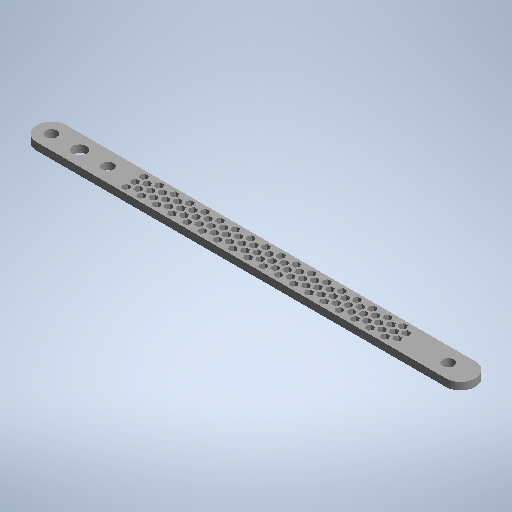
# Autodesk Inventor part: RT_ARM_PR_001
Saved by Autodesk Inventor 2025.4 (Build 294407000, 407)
## iProperties
Created: 2026-04-27
Part Number: RT_ARM_PR_001
Material: Générique
Document SubType Name: Modeling
Designer: louis
Density: 1 g/cm^3
Appearance: Par défaut
Author: louis
Autodesk Inventor part; units mm, degrees
ref_plane "YZ Plane" through (0, 0, 0) normal (1, 0, 0) x (0, 1, 0)
ref_plane "XZ Plane" through (0, 0, 0) normal (0, 1, 0) x (-1, 0, 0)
ref_plane "XY Plane" through (0, 0, 0) normal (0, 0, 1) x (1, 0, 0)
sketch "Sketch2" plane through (0, 0, 0) normal (0, 0, 1) x (1, 0, 0)
  line L0 (-89.25, 6) -> (89.25, 6)
  line L1 (89.25, 6) -> (89.25, -6)
  line L2 (89.25, -6) -> (-89.25, -6)
  line L3 (-89.25, -6) -> (-89.25, 6)
  line L4 (-89.25, 6) -> (89.25, -6) construction
  line L5 (89.25, 6) -> (-89.25, -6) construction
  line L6 (-83.25, 0) -> (-60.25, 0) construction
  line L7 (-83.25, -6) -> (-60.25, -6)
  line L8 (-60.25, 6) -> (-83.25, 6)
  arc A0 (-83.25, 6) -> (-83.25, -6) centre (-83.25, 0) ccw
  arc A1 (-60.25, -6) -> (-60.25, 6) centre (-60.25, 0) ccw
  line L9 (73.25, 0) -> (83.25, 0) construction
  line L10 (73.25, -6) -> (83.25, -6)
  line L11 (83.25, 6) -> (73.25, 6)
  arc A2 (73.25, 6) -> (73.25, -6) centre (73.25, 0) ccw
  arc A3 (83.25, -6) -> (83.25, 6) centre (83.25, 0) ccw
  line L12 (-47.75, 0) -> (-48.5, -1.299)
  line L13 (-48.5, -1.299) -> (-50, -1.299)
  line L14 (-50, -1.299) -> (-50.75, 0)
  line L15 (-50.75, 0) -> (-50, 1.299)
  line L16 (-50, 1.299) -> (-48.5, 1.299)
  line L17 (-48.5, 1.299) -> (-47.75, 0)
  line L18 (-47.75, 3.5981) -> (-48.5, 2.299)
  line L19 (-48.5, 2.299) -> (-50, 2.299)
  line L20 (-50, 2.299) -> (-50.75, 3.5981)
  line L21 (-50.75, 3.5981) -> (-50, 4.8971)
  line L22 (-50, 4.8971) -> (-48.5, 4.8971)
  line L23 (-48.5, 4.8971) -> (-47.75, 3.5981)
  line L24 (-50, 1.299) -> (-50, 2.299) construction
  line L25 (-45.384, 0.5) -> (-46.884, 0.5)
  line L26 (-46.884, 0.5) -> (-47.634, 1.799)
  line L27 (-47.634, 1.799) -> (-46.884, 3.0981)
  line L28 (-46.884, 3.0981) -> (-45.384, 3.0981)
  line L29 (-45.384, 3.0981) -> (-44.634, 1.799)
  line L30 (-44.634, 1.799) -> (-45.384, 0.5)
  line L31 (-48.5, -4.8971) -> (-50, -4.8971)
  line L32 (-50, -4.8971) -> (-50.75, -3.5981)
  line L33 (-50.75, -3.5981) -> (-50, -2.299)
  line L34 (-50, -2.299) -> (-48.5, -2.299)
  line L35 (-48.5, -2.299) -> (-47.75, -3.5981)
  line L36 (-47.75, -3.5981) -> (-48.5, -4.8971)
  line L37 (-44.634, -1.799) -> (-45.384, -3.0981)
  line L38 (-45.384, -3.0981) -> (-46.884, -3.0981)
  line L39 (-46.884, -3.0981) -> (-47.634, -1.799)
  line L40 (-47.634, -1.799) -> (-46.884, -0.5)
  line L41 (-46.884, -0.5) -> (-45.384, -0.5)
  line L42 (-45.384, -0.5) -> (-44.634, -1.799)
  line L43 (-50, -1.299) -> (-50, -2.299) construction
  line L44 (-44.634, 1.799) -> (-43.7679, 2.299) construction
  line L45 (-43.7679, 2.299) -> (-43.7679, 1.299) construction
  line L46 (-43.7679, 1.299) -> (-44.634, 1.799) construction
  line L47 (-43.7679, 1.299) -> (-44.5179, 0) construction
  line L48 (-44.5179, 0) -> (-45.384, 0.5) construction
  line L49 (-45.384, -0.5) -> (-44.5179, 0) construction
  line L50 (-50.75, 3.5981) -> (-50.75, 0) construction
  line L51 (-44.55, 3.5981) -> (-44.55, 0) construction
  line L52 (-44.55, 0) -> (-43.8, 1.299)
  line L53 (-44.55, 3.5981) -> (-43.8, 4.8971)
  line L54 (-43.8, 2.299) -> (-44.55, 3.5981)
  line L55 (-43.8, 1.299) -> (-43.8, 2.299) construction
  line L56 (-42.3, 2.299) -> (-43.8, 2.299)
  line L57 (-43.8, 4.8971) -> (-42.3, 4.8971)
  line L58 (-43.8, 1.299) -> (-42.3, 1.299)
  line L59 (-42.3, 1.299) -> (-41.55, 0)
  line L60 (-41.55, 3.5981) -> (-42.3, 2.299)
  line L61 (-40.684, 0.5) -> (-41.434, 1.799)
  line L62 (-41.434, 1.799) -> (-40.684, 3.0981)
  line L63 (-42.3, 4.8971) -> (-41.55, 3.5981)
  line L64 (-41.55, 0) -> (-42.3, -1.299)
  line L65 (-42.3, -1.299) -> (-43.8, -1.299)
  line L66 (-43.8, -1.299) -> (-44.55, 0)
  line L67 (-43.8, -1.299) -> (-43.8, -2.299) construction
  line L68 (-43.8, -2.299) -> (-42.3, -2.299)
  line L69 (-40.684, -3.0981) -> (-41.434, -1.799)
  line L70 (-44.55, -3.5981) -> (-43.8, -2.299)
  line L71 (-42.3, -2.299) -> (-41.55, -3.5981)
  line L72 (-43.8, -4.8971) -> (-44.55, -3.5981)
  line L73 (-42.3, -4.8971) -> (-43.8, -4.8971)
  line L74 (-41.55, -3.5981) -> (-42.3, -4.8971)
  line L75 (-41.434, -1.799) -> (-40.684, -0.5)
  line L76 (-38.3179, 0) -> (-39.184, 0.5) construction
  line L77 (-39.184, -0.5) -> (-38.3179, 0) construction
  line L78 (-39.184, 3.0981) -> (-38.434, 1.799)
  line L79 (-38.434, 1.799) -> (-39.184, 0.5)
  line L80 (-38.434, -1.799) -> (-39.184, -3.0981)
  line L81 (-39.184, -0.5) -> (-38.434, -1.799)
  line L82 (-39.184, -3.0981) -> (-40.684, -3.0981)
  line L83 (-40.684, -0.5) -> (-39.184, -0.5)
  line L84 (-39.184, 0.5) -> (-40.684, 0.5)
  line L85 (-40.684, 3.0981) -> (-39.184, 3.0981)
  line L86 (-38.35, 3.5981) -> (-38.35, 0) construction
  line L87 (-38.35, 0) -> (-37.6, 1.299)
  line L88 (-38.35, 3.5981) -> (-37.6, 4.8971)
  line L89 (-37.6, 2.299) -> (-38.35, 3.5981)
  line L90 (-37.6, 1.299) -> (-37.6, 2.299) construction
  line L91 (-36.1, 2.299) -> (-37.6, 2.299)
  line L92 (-37.6, 4.8971) -> (-36.1, 4.8971)
  line L93 (-37.6, 1.299) -> (-36.1, 1.299)
  line L94 (-36.1, 1.299) -> (-35.35, 0)
  line L95 (-35.35, 3.5981) -> (-36.1, 2.299)
  line L96 (-34.484, 0.5) -> (-35.234, 1.799)
  line L97 (-35.234, 1.799) -> (-34.484, 3.0981)
  line L98 (-36.1, 4.8971) -> (-35.35, 3.5981)
  line L99 (-35.35, 0) -> (-36.1, -1.299)
  line L100 (-36.1, -1.299) -> (-37.6, -1.299)
  line L101 (-37.6, -1.299) -> (-38.35, 0)
  line L102 (-37.6, -1.299) -> (-37.6, -2.299) construction
  line L103 (-37.6, -2.299) -> (-36.1, -2.299)
  line L104 (-34.484, -3.0981) -> (-35.234, -1.799)
  line L105 (-38.35, -3.5981) -> (-37.6, -2.299)
  line L106 (-36.1, -2.299) -> (-35.35, -3.5981)
  line L107 (-37.6, -4.8971) -> (-38.35, -3.5981)
  line L108 (-36.1, -4.8971) -> (-37.6, -4.8971)
  line L109 (-35.35, -3.5981) -> (-36.1, -4.8971)
  line L110 (-35.234, -1.799) -> (-34.484, -0.5)
  line L111 (-32.1179, 0) -> (-32.984, 0.5) construction
  line L112 (-32.984, -0.5) -> (-32.1179, 0) construction
  line L113 (-32.984, 3.0981) -> (-32.234, 1.799)
  line L114 (-32.234, 1.799) -> (-32.984, 0.5)
  line L115 (-32.234, -1.799) -> (-32.984, -3.0981)
  line L116 (-32.984, -0.5) -> (-32.234, -1.799)
  line L117 (-32.984, -3.0981) -> (-34.484, -3.0981)
  line L118 (-34.484, -0.5) -> (-32.984, -0.5)
  line L119 (-32.984, 0.5) -> (-34.484, 0.5)
  line L120 (-34.484, 3.0981) -> (-32.984, 3.0981)
  line L121 (-32.15, 3.5981) -> (-32.15, 0) construction
  line L122 (-32.15, 0) -> (-31.4, 1.299)
  line L123 (-32.15, 3.5981) -> (-31.4, 4.8971)
  line L124 (-31.4, 2.299) -> (-32.15, 3.5981)
  line L125 (-31.4, 1.299) -> (-31.4, 2.299) construction
  line L126 (-29.9, 2.299) -> (-31.4, 2.299)
  line L127 (-31.4, 4.8971) -> (-29.9, 4.8971)
  line L128 (-31.4, 1.299) -> (-29.9, 1.299)
  line L129 (-29.9, 1.299) -> (-29.15, 0)
  line L130 (-29.15, 3.5981) -> (-29.9, 2.299)
  line L131 (-28.284, 0.5) -> (-29.034, 1.799)
  line L132 (-29.034, 1.799) -> (-28.284, 3.0981)
  line L133 (-29.9, 4.8971) -> (-29.15, 3.5981)
  line L134 (-29.15, 0) -> (-29.9, -1.299)
  line L135 (-29.9, -1.299) -> (-31.4, -1.299)
  line L136 (-31.4, -1.299) -> (-32.15, 0)
  line L137 (-31.4, -1.299) -> (-31.4, -2.299) construction
  line L138 (-31.4, -2.299) -> (-29.9, -2.299)
  line L139 (-28.284, -3.0981) -> (-29.034, -1.799)
  line L140 (-32.15, -3.5981) -> (-31.4, -2.299)
  line L141 (-29.9, -2.299) -> (-29.15, -3.5981)
  line L142 (-31.4, -4.8971) -> (-32.15, -3.5981)
  line L143 (-29.9, -4.8971) -> (-31.4, -4.8971)
  line L144 (-29.15, -3.5981) -> (-29.9, -4.8971)
  line L145 (-29.034, -1.799) -> (-28.284, -0.5)
  line L146 (-25.9179, 0) -> (-26.784, 0.5) construction
  line L147 (-26.784, -0.5) -> (-25.9179, 0) construction
  line L148 (-26.784, 3.0981) -> (-26.034, 1.799)
  line L149 (-26.034, 1.799) -> (-26.784, 0.5)
  line L150 (-26.034, -1.799) -> (-26.784, -3.0981)
  line L151 (-26.784, -0.5) -> (-26.034, -1.799)
  line L152 (-26.784, -3.0981) -> (-28.284, -3.0981)
  line L153 (-28.284, -0.5) -> (-26.784, -0.5)
  line L154 (-26.784, 0.5) -> (-28.284, 0.5)
  line L155 (-28.284, 3.0981) -> (-26.784, 3.0981)
  line L156 (-25.95, 3.5981) -> (-25.95, 0) construction
  line L157 (-25.95, 0) -> (-25.2, 1.299)
  line L158 (-25.95, 3.5981) -> (-25.2, 4.8971)
  line L159 (-25.2, 2.299) -> (-25.95, 3.5981)
  line L160 (-25.2, 1.299) -> (-25.2, 2.299) construction
  line L161 (-23.7, 2.299) -> (-25.2, 2.299)
  line L162 (-25.2, 4.8971) -> (-23.7, 4.8971)
  line L163 (-25.2, 1.299) -> (-23.7, 1.299)
  line L164 (-23.7, 1.299) -> (-22.95, 0)
  line L165 (-22.95, 3.5981) -> (-23.7, 2.299)
  line L166 (-22.084, 0.5) -> (-22.834, 1.799)
  line L167 (-22.834, 1.799) -> (-22.084, 3.0981)
  line L168 (-23.7, 4.8971) -> (-22.95, 3.5981)
  line L169 (-22.95, 0) -> (-23.7, -1.299)
  line L170 (-23.7, -1.299) -> (-25.2, -1.299)
  line L171 (-25.2, -1.299) -> (-25.95, 0)
  line L172 (-25.2, -1.299) -> (-25.2, -2.299) construction
  line L173 (-25.2, -2.299) -> (-23.7, -2.299)
  line L174 (-22.084, -3.0981) -> (-22.834, -1.799)
  line L175 (-25.95, -3.5981) -> (-25.2, -2.299)
  line L176 (-23.7, -2.299) -> (-22.95, -3.5981)
  line L177 (-25.2, -4.8971) -> (-25.95, -3.5981)
  line L178 (-23.7, -4.8971) -> (-25.2, -4.8971)
  line L179 (-22.95, -3.5981) -> (-23.7, -4.8971)
  line L180 (-22.834, -1.799) -> (-22.084, -0.5)
  line L181 (-19.7179, 0) -> (-20.584, 0.5) construction
  line L182 (-20.584, -0.5) -> (-19.7179, 0) construction
  line L183 (-20.584, 3.0981) -> (-19.834, 1.799)
  line L184 (-19.834, 1.799) -> (-20.584, 0.5)
  line L185 (-19.834, -1.799) -> (-20.584, -3.0981)
  line L186 (-20.584, -0.5) -> (-19.834, -1.799)
  line L187 (-20.584, -3.0981) -> (-22.084, -3.0981)
  line L188 (-22.084, -0.5) -> (-20.584, -0.5)
  line L189 (-20.584, 0.5) -> (-22.084, 0.5)
  line L190 (-22.084, 3.0981) -> (-20.584, 3.0981)
  line L191 (-19.75, 3.5981) -> (-19.75, 0) construction
  line L192 (-19.75, 0) -> (-19, 1.299)
  line L193 (-19.75, 3.5981) -> (-19, 4.8971)
  line L194 (-19, 2.299) -> (-19.75, 3.5981)
  line L195 (-19, 1.299) -> (-19, 2.299) construction
  line L196 (-17.5, 2.299) -> (-19, 2.299)
  line L197 (-19, 4.8971) -> (-17.5, 4.8971)
  line L198 (-19, 1.299) -> (-17.5, 1.299)
  line L199 (-17.5, 1.299) -> (-16.75, 0)
  line L200 (-16.75, 3.5981) -> (-17.5, 2.299)
  line L201 (-15.884, 0.5) -> (-16.634, 1.799)
  line L202 (-16.634, 1.799) -> (-15.884, 3.0981)
  line L203 (-17.5, 4.8971) -> (-16.75, 3.5981)
  line L204 (-16.75, 0) -> (-17.5, -1.299)
  line L205 (-17.5, -1.299) -> (-19, -1.299)
  line L206 (-19, -1.299) -> (-19.75, 0)
  line L207 (-19, -1.299) -> (-19, -2.299) construction
  line L208 (-19, -2.299) -> (-17.5, -2.299)
  line L209 (-15.884, -3.0981) -> (-16.634, -1.799)
  line L210 (-19.75, -3.5981) -> (-19, -2.299)
  line L211 (-17.5, -2.299) -> (-16.75, -3.5981)
  line L212 (-19, -4.8971) -> (-19.75, -3.5981)
  line L213 (-17.5, -4.8971) -> (-19, -4.8971)
  line L214 (-16.75, -3.5981) -> (-17.5, -4.8971)
  line L215 (-16.634, -1.799) -> (-15.884, -0.5)
  line L216 (-13.5179, 0) -> (-14.384, 0.5) construction
  line L217 (-14.384, -0.5) -> (-13.5179, 0) construction
  line L218 (-14.384, 3.0981) -> (-13.634, 1.799)
  line L219 (-13.634, 1.799) -> (-14.384, 0.5)
  line L220 (-13.634, -1.799) -> (-14.384, -3.0981)
  line L221 (-14.384, -0.5) -> (-13.634, -1.799)
  line L222 (-14.384, -3.0981) -> (-15.884, -3.0981)
  line L223 (-15.884, -0.5) -> (-14.384, -0.5)
  line L224 (-14.384, 0.5) -> (-15.884, 0.5)
  line L225 (-15.884, 3.0981) -> (-14.384, 3.0981)
  line L226 (-13.55, 3.5981) -> (-13.55, 0) construction
  line L227 (-13.55, 0) -> (-12.8, 1.299)
  line L228 (-13.55, 3.5981) -> (-12.8, 4.8971)
  line L229 (-12.8, 2.299) -> (-13.55, 3.5981)
  line L230 (-12.8, 1.299) -> (-12.8, 2.299) construction
  line L231 (-11.3, 2.299) -> (-12.8, 2.299)
  line L232 (-12.8, 4.8971) -> (-11.3, 4.8971)
  line L233 (-12.8, 1.299) -> (-11.3, 1.299)
  line L234 (-11.3, 1.299) -> (-10.55, 0)
  line L235 (-10.55, 3.5981) -> (-11.3, 2.299)
  line L236 (-9.684, 0.5) -> (-10.434, 1.799)
  line L237 (-10.434, 1.799) -> (-9.684, 3.0981)
  line L238 (-11.3, 4.8971) -> (-10.55, 3.5981)
  line L239 (-10.55, 0) -> (-11.3, -1.299)
  line L240 (-11.3, -1.299) -> (-12.8, -1.299)
  line L241 (-12.8, -1.299) -> (-13.55, 0)
  line L242 (-12.8, -1.299) -> (-12.8, -2.299) construction
  line L243 (-12.8, -2.299) -> (-11.3, -2.299)
  line L244 (-9.684, -3.0981) -> (-10.434, -1.799)
  line L245 (-13.55, -3.5981) -> (-12.8, -2.299)
  line L246 (-11.3, -2.299) -> (-10.55, -3.5981)
  line L247 (-12.8, -4.8971) -> (-13.55, -3.5981)
  line L248 (-11.3, -4.8971) -> (-12.8, -4.8971)
  line L249 (-10.55, -3.5981) -> (-11.3, -4.8971)
  line L250 (-10.434, -1.799) -> (-9.684, -0.5)
  line L251 (-7.3179, 0) -> (-8.184, 0.5) construction
  line L252 (-8.184, -0.5) -> (-7.3179, 0) construction
  line L253 (-8.184, 3.0981) -> (-7.434, 1.799)
  line L254 (-7.434, 1.799) -> (-8.184, 0.5)
  line L255 (-7.434, -1.799) -> (-8.184, -3.0981)
  line L256 (-8.184, -0.5) -> (-7.434, -1.799)
  line L257 (-8.184, -3.0981) -> (-9.684, -3.0981)
  line L258 (-9.684, -0.5) -> (-8.184, -0.5)
  line L259 (-8.184, 0.5) -> (-9.684, 0.5)
  line L260 (-9.684, 3.0981) -> (-8.184, 3.0981)
  line L261 (-7.35, 3.5981) -> (-7.35, 0) construction
  line L262 (-7.35, 0) -> (-6.6, 1.299)
  line L263 (-7.35, 3.5981) -> (-6.6, 4.8971)
  line L264 (-6.6, 2.299) -> (-7.35, 3.5981)
  line L265 (-6.6, 1.299) -> (-6.6, 2.299) construction
  line L266 (-5.1, 2.299) -> (-6.6, 2.299)
  line L267 (-6.6, 4.8971) -> (-5.1, 4.8971)
  line L268 (-6.6, 1.299) -> (-5.1, 1.299)
  line L269 (-5.1, 1.299) -> (-4.35, 0)
  line L270 (-4.35, 3.5981) -> (-5.1, 2.299)
  line L271 (-3.484, 0.5) -> (-4.234, 1.799)
  line L272 (-4.234, 1.799) -> (-3.484, 3.0981)
  line L273 (-5.1, 4.8971) -> (-4.35, 3.5981)
  line L274 (-4.35, 0) -> (-5.1, -1.299)
  line L275 (-5.1, -1.299) -> (-6.6, -1.299)
  line L276 (-6.6, -1.299) -> (-7.35, 0)
  line L277 (-6.6, -1.299) -> (-6.6, -2.299) construction
  line L278 (-6.6, -2.299) -> (-5.1, -2.299)
  line L279 (-3.484, -3.0981) -> (-4.234, -1.799)
  line L280 (-7.35, -3.5981) -> (-6.6, -2.299)
  line L281 (-5.1, -2.299) -> (-4.35, -3.5981)
  line L282 (-6.6, -4.8971) -> (-7.35, -3.5981)
  line L283 (-5.1, -4.8971) -> (-6.6, -4.8971)
  line L284 (-4.35, -3.5981) -> (-5.1, -4.8971)
  line L285 (-4.234, -1.799) -> (-3.484, -0.5)
  line L286 (-1.1179, 0) -> (-1.984, 0.5) construction
  line L287 (-1.984, -0.5) -> (-1.1179, 0) construction
  line L288 (-1.984, 3.0981) -> (-1.234, 1.799)
  line L289 (-1.234, 1.799) -> (-1.984, 0.5)
  line L290 (-1.234, -1.799) -> (-1.984, -3.0981)
  line L291 (-1.984, -0.5) -> (-1.234, -1.799)
  line L292 (-1.984, -3.0981) -> (-3.484, -3.0981)
  line L293 (-3.484, -0.5) -> (-1.984, -0.5)
  line L294 (-1.984, 0.5) -> (-3.484, 0.5)
  line L295 (-3.484, 3.0981) -> (-1.984, 3.0981)
  line L296 (-1.15, 3.5981) -> (-1.15, 0) construction
  line L297 (-1.15, 0) -> (-0.4, 1.299)
  line L298 (-1.15, 3.5981) -> (-0.4, 4.8971)
  line L299 (-0.4, 2.299) -> (-1.15, 3.5981)
  line L300 (-0.4, 1.299) -> (-0.4, 2.299) construction
  line L301 (1.1, 2.299) -> (-0.4, 2.299)
  line L302 (-0.4, 4.8971) -> (1.1, 4.8971)
  line L303 (-0.4, 1.299) -> (1.1, 1.299)
  line L304 (1.1, 1.299) -> (1.85, 0)
  line L305 (1.85, 3.5981) -> (1.1, 2.299)
  line L306 (2.716, 0.5) -> (1.966, 1.799)
  line L307 (1.966, 1.799) -> (2.716, 3.0981)
  line L308 (1.1, 4.8971) -> (1.85, 3.5981)
  line L309 (1.85, 0) -> (1.1, -1.299)
  line L310 (1.1, -1.299) -> (-0.4, -1.299)
  line L311 (-0.4, -1.299) -> (-1.15, 0)
  line L312 (-0.4, -1.299) -> (-0.4, -2.299) construction
  line L313 (-0.4, -2.299) -> (1.1, -2.299)
  line L314 (2.716, -3.0981) -> (1.966, -1.799)
  line L315 (-1.15, -3.5981) -> (-0.4, -2.299)
  line L316 (1.1, -2.299) -> (1.85, -3.5981)
  line L317 (-0.4, -4.8971) -> (-1.15, -3.5981)
  line L318 (1.1, -4.8971) -> (-0.4, -4.8971)
  line L319 (1.85, -3.5981) -> (1.1, -4.8971)
  line L320 (1.966, -1.799) -> (2.716, -0.5)
  line L321 (5.0821, 0) -> (4.216, 0.5) construction
  line L322 (4.216, -0.5) -> (5.0821, 0) construction
  line L323 (4.216, 3.0981) -> (4.966, 1.799)
  line L324 (4.966, 1.799) -> (4.216, 0.5)
  line L325 (4.966, -1.799) -> (4.216, -3.0981)
  line L326 (4.216, -0.5) -> (4.966, -1.799)
  line L327 (4.216, -3.0981) -> (2.716, -3.0981)
  line L328 (2.716, -0.5) -> (4.216, -0.5)
  line L329 (4.216, 0.5) -> (2.716, 0.5)
  line L330 (2.716, 3.0981) -> (4.216, 3.0981)
  line L331 (5.05, 3.5981) -> (5.05, 0) construction
  line L332 (5.05, 0) -> (5.8, 1.299)
  line L333 (5.05, 3.5981) -> (5.8, 4.8971)
  line L334 (5.8, 2.299) -> (5.05, 3.5981)
  line L335 (5.8, 1.299) -> (5.8, 2.299) construction
  line L336 (7.3, 2.299) -> (5.8, 2.299)
  line L337 (5.8, 4.8971) -> (7.3, 4.8971)
  line L338 (5.8, 1.299) -> (7.3, 1.299)
  line L339 (7.3, 1.299) -> (8.05, 0)
  line L340 (8.05, 3.5981) -> (7.3, 2.299)
  line L341 (8.916, 0.5) -> (8.166, 1.799)
  line L342 (8.166, 1.799) -> (8.916, 3.0981)
  line L343 (7.3, 4.8971) -> (8.05, 3.5981)
  line L344 (8.05, 0) -> (7.3, -1.299)
  line L345 (7.3, -1.299) -> (5.8, -1.299)
  line L346 (5.8, -1.299) -> (5.05, 0)
  line L347 (5.8, -1.299) -> (5.8, -2.299) construction
  line L348 (5.8, -2.299) -> (7.3, -2.299)
  line L349 (8.916, -3.0981) -> (8.166, -1.799)
  line L350 (5.05, -3.5981) -> (5.8, -2.299)
  line L351 (7.3, -2.299) -> (8.05, -3.5981)
  line L352 (5.8, -4.8971) -> (5.05, -3.5981)
  line L353 (7.3, -4.8971) -> (5.8, -4.8971)
  line L354 (8.05, -3.5981) -> (7.3, -4.8971)
  line L355 (8.166, -1.799) -> (8.916, -0.5)
  line L356 (11.2821, 0) -> (10.416, 0.5) construction
  line L357 (10.416, -0.5) -> (11.2821, 0) construction
  line L358 (10.416, 3.0981) -> (11.166, 1.799)
  line L359 (11.166, 1.799) -> (10.416, 0.5)
  line L360 (11.166, -1.799) -> (10.416, -3.0981)
  line L361 (10.416, -0.5) -> (11.166, -1.799)
  line L362 (10.416, -3.0981) -> (8.916, -3.0981)
  line L363 (8.916, -0.5) -> (10.416, -0.5)
  line L364 (10.416, 0.5) -> (8.916, 0.5)
  line L365 (8.916, 3.0981) -> (10.416, 3.0981)
  line L366 (11.25, 3.5981) -> (11.25, 0) construction
  line L367 (11.25, 0) -> (12, 1.299)
  line L368 (11.25, 3.5981) -> (12, 4.8971)
  line L369 (12, 2.299) -> (11.25, 3.5981)
  line L370 (12, 1.299) -> (12, 2.299) construction
  line L371 (13.5, 2.299) -> (12, 2.299)
  line L372 (12, 4.8971) -> (13.5, 4.8971)
  line L373 (12, 1.299) -> (13.5, 1.299)
  line L374 (13.5, 1.299) -> (14.25, 0)
  line L375 (14.25, 3.5981) -> (13.5, 2.299)
  line L376 (15.116, 0.5) -> (14.366, 1.799)
  line L377 (14.366, 1.799) -> (15.116, 3.0981)
  line L378 (13.5, 4.8971) -> (14.25, 3.5981)
  line L379 (14.25, 0) -> (13.5, -1.299)
  line L380 (13.5, -1.299) -> (12, -1.299)
  line L381 (12, -1.299) -> (11.25, 0)
  line L382 (12, -1.299) -> (12, -2.299) construction
  line L383 (12, -2.299) -> (13.5, -2.299)
  line L384 (15.116, -3.0981) -> (14.366, -1.799)
  line L385 (11.25, -3.5981) -> (12, -2.299)
  line L386 (13.5, -2.299) -> (14.25, -3.5981)
  line L387 (12, -4.8971) -> (11.25, -3.5981)
  line L388 (13.5, -4.8971) -> (12, -4.8971)
  line L389 (14.25, -3.5981) -> (13.5, -4.8971)
  line L390 (14.366, -1.799) -> (15.116, -0.5)
  line L391 (17.4821, 0) -> (16.616, 0.5) construction
  line L392 (16.616, -0.5) -> (17.4821, 0) construction
  line L393 (16.616, 3.0981) -> (17.366, 1.799)
  line L394 (17.366, 1.799) -> (16.616, 0.5)
  line L395 (17.366, -1.799) -> (16.616, -3.0981)
  line L396 (16.616, -0.5) -> (17.366, -1.799)
  line L397 (16.616, -3.0981) -> (15.116, -3.0981)
  line L398 (15.116, -0.5) -> (16.616, -0.5)
  line L399 (16.616, 0.5) -> (15.116, 0.5)
  line L400 (15.116, 3.0981) -> (16.616, 3.0981)
  line L401 (17.45, 3.5981) -> (17.45, 0) construction
  line L402 (17.45, 0) -> (18.2, 1.299)
  line L403 (17.45, 3.5981) -> (18.2, 4.8971)
  line L404 (18.2, 2.299) -> (17.45, 3.5981)
  line L405 (18.2, 1.299) -> (18.2, 2.299) construction
  line L406 (19.7, 2.299) -> (18.2, 2.299)
  line L407 (18.2, 4.8971) -> (19.7, 4.8971)
  line L408 (18.2, 1.299) -> (19.7, 1.299)
  line L409 (19.7, 1.299) -> (20.45, 0)
  line L410 (20.45, 3.5981) -> (19.7, 2.299)
  line L411 (21.316, 0.5) -> (20.566, 1.799)
  line L412 (20.566, 1.799) -> (21.316, 3.0981)
  line L413 (19.7, 4.8971) -> (20.45, 3.5981)
  line L414 (20.45, 0) -> (19.7, -1.299)
  line L415 (19.7, -1.299) -> (18.2, -1.299)
  line L416 (18.2, -1.299) -> (17.45, 0)
  line L417 (18.2, -1.299) -> (18.2, -2.299) construction
  line L418 (18.2, -2.299) -> (19.7, -2.299)
  line L419 (21.316, -3.0981) -> (20.566, -1.799)
  line L420 (17.45, -3.5981) -> (18.2, -2.299)
  line L421 (19.7, -2.299) -> (20.45, -3.5981)
  line L422 (18.2, -4.8971) -> (17.45, -3.5981)
  line L423 (19.7, -4.8971) -> (18.2, -4.8971)
  line L424 (20.45, -3.5981) -> (19.7, -4.8971)
  line L425 (20.566, -1.799) -> (21.316, -0.5)
  line L426 (23.6821, 0) -> (22.816, 0.5) construction
  line L427 (22.816, -0.5) -> (23.6821, 0) construction
  line L428 (22.816, 3.0981) -> (23.566, 1.799)
  line L429 (23.566, 1.799) -> (22.816, 0.5)
  line L430 (23.566, -1.799) -> (22.816, -3.0981)
  line L431 (22.816, -0.5) -> (23.566, -1.799)
  line L432 (22.816, -3.0981) -> (21.316, -3.0981)
  line L433 (21.316, -0.5) -> (22.816, -0.5)
  line L434 (22.816, 0.5) -> (21.316, 0.5)
  line L435 (21.316, 3.0981) -> (22.816, 3.0981)
  line L436 (23.65, 3.5981) -> (23.65, 0) construction
  line L437 (23.65, 0) -> (24.4, 1.299)
  line L438 (23.65, 3.5981) -> (24.4, 4.8971)
  line L439 (24.4, 2.299) -> (23.65, 3.5981)
  line L440 (24.4, 1.299) -> (24.4, 2.299) construction
  line L441 (25.9, 2.299) -> (24.4, 2.299)
  line L442 (24.4, 4.8971) -> (25.9, 4.8971)
  line L443 (24.4, 1.299) -> (25.9, 1.299)
  line L444 (25.9, 1.299) -> (26.65, 0)
  line L445 (26.65, 3.5981) -> (25.9, 2.299)
  line L446 (27.516, 0.5) -> (26.766, 1.799)
  line L447 (26.766, 1.799) -> (27.516, 3.0981)
  line L448 (25.9, 4.8971) -> (26.65, 3.5981)
  line L449 (26.65, 0) -> (25.9, -1.299)
  line L450 (25.9, -1.299) -> (24.4, -1.299)
  line L451 (24.4, -1.299) -> (23.65, 0)
  line L452 (24.4, -1.299) -> (24.4, -2.299) construction
  line L453 (24.4, -2.299) -> (25.9, -2.299)
  line L454 (27.516, -3.0981) -> (26.766, -1.799)
  line L455 (23.65, -3.5981) -> (24.4, -2.299)
  line L456 (25.9, -2.299) -> (26.65, -3.5981)
  line L457 (24.4, -4.8971) -> (23.65, -3.5981)
  line L458 (25.9, -4.8971) -> (24.4, -4.8971)
  line L459 (26.65, -3.5981) -> (25.9, -4.8971)
  line L460 (26.766, -1.799) -> (27.516, -0.5)
  line L461 (29.8821, 0) -> (29.016, 0.5) construction
  line L462 (29.016, -0.5) -> (29.8821, 0) construction
  line L463 (29.016, 3.0981) -> (29.766, 1.799)
  line L464 (29.766, 1.799) -> (29.016, 0.5)
  line L465 (29.766, -1.799) -> (29.016, -3.0981)
  line L466 (29.016, -0.5) -> (29.766, -1.799)
  line L467 (29.016, -3.0981) -> (27.516, -3.0981)
  line L468 (27.516, -0.5) -> (29.016, -0.5)
  line L469 (29.016, 0.5) -> (27.516, 0.5)
  line L470 (27.516, 3.0981) -> (29.016, 3.0981)
  line L471 (29.85, 3.5981) -> (29.85, 0) construction
  line L472 (29.85, 0) -> (30.6, 1.299)
  line L473 (29.85, 3.5981) -> (30.6, 4.8971)
  line L474 (30.6, 2.299) -> (29.85, 3.5981)
  line L475 (30.6, 1.299) -> (30.6, 2.299) construction
  line L476 (32.1, 2.299) -> (30.6, 2.299)
  line L477 (30.6, 4.8971) -> (32.1, 4.8971)
  line L478 (30.6, 1.299) -> (32.1, 1.299)
  line L479 (32.1, 1.299) -> (32.85, 0)
  line L480 (32.85, 3.5981) -> (32.1, 2.299)
  line L481 (33.716, 0.5) -> (32.966, 1.799)
  line L482 (32.966, 1.799) -> (33.716, 3.0981)
  line L483 (32.1, 4.8971) -> (32.85, 3.5981)
  line L484 (32.85, 0) -> (32.1, -1.299)
  line L485 (32.1, -1.299) -> (30.6, -1.299)
  line L486 (30.6, -1.299) -> (29.85, 0)
  line L487 (30.6, -1.299) -> (30.6, -2.299) construction
  line L488 (30.6, -2.299) -> (32.1, -2.299)
  line L489 (33.716, -3.0981) -> (32.966, -1.799)
  line L490 (29.85, -3.5981) -> (30.6, -2.299)
  line L491 (32.1, -2.299) -> (32.85, -3.5981)
  line L492 (30.6, -4.8971) -> (29.85, -3.5981)
  line L493 (32.1, -4.8971) -> (30.6, -4.8971)
  line L494 (32.85, -3.5981) -> (32.1, -4.8971)
  line L495 (32.966, -1.799) -> (33.716, -0.5)
  line L496 (36.0821, 0) -> (35.216, 0.5) construction
  line L497 (35.216, -0.5) -> (36.0821, 0) construction
  line L498 (35.216, 3.0981) -> (35.966, 1.799)
  line L499 (35.966, 1.799) -> (35.216, 0.5)
  line L500 (35.966, -1.799) -> (35.216, -3.0981)
  line L501 (35.216, -0.5) -> (35.966, -1.799)
  line L502 (35.216, -3.0981) -> (33.716, -3.0981)
  line L503 (33.716, -0.5) -> (35.216, -0.5)
  line L504 (35.216, 0.5) -> (33.716, 0.5)
  line L505 (33.716, 3.0981) -> (35.216, 3.0981)
  line L506 (36.05, 3.5981) -> (36.05, 0) construction
  line L507 (36.05, 0) -> (36.8, 1.299)
  line L508 (36.05, 3.5981) -> (36.8, 4.8971)
  line L509 (36.8, 2.299) -> (36.05, 3.5981)
  line L510 (36.8, 1.299) -> (36.8, 2.299) construction
  line L511 (38.3, 2.299) -> (36.8, 2.299)
  line L512 (36.8, 4.8971) -> (38.3, 4.8971)
  line L513 (36.8, 1.299) -> (38.3, 1.299)
  line L514 (38.3, 1.299) -> (39.05, 0)
  line L515 (39.05, 3.5981) -> (38.3, 2.299)
  line L516 (39.916, 0.5) -> (39.166, 1.799)
  line L517 (39.166, 1.799) -> (39.916, 3.0981)
  line L518 (38.3, 4.8971) -> (39.05, 3.5981)
  line L519 (39.05, 0) -> (38.3, -1.299)
  line L520 (38.3, -1.299) -> (36.8, -1.299)
  line L521 (36.8, -1.299) -> (36.05, 0)
  line L522 (36.8, -1.299) -> (36.8, -2.299) construction
  line L523 (36.8, -2.299) -> (38.3, -2.299)
  line L524 (39.916, -3.0981) -> (39.166, -1.799)
  line L525 (36.05, -3.5981) -> (36.8, -2.299)
  line L526 (38.3, -2.299) -> (39.05, -3.5981)
  line L527 (36.8, -4.8971) -> (36.05, -3.5981)
  line L528 (38.3, -4.8971) -> (36.8, -4.8971)
  line L529 (39.05, -3.5981) -> (38.3, -4.8971)
  line L530 (39.166, -1.799) -> (39.916, -0.5)
  line L531 (42.2821, 0) -> (41.416, 0.5) construction
  line L532 (41.416, -0.5) -> (42.2821, 0) construction
  line L533 (41.416, 3.0981) -> (42.166, 1.799)
  line L534 (42.166, 1.799) -> (41.416, 0.5)
  line L535 (42.166, -1.799) -> (41.416, -3.0981)
  line L536 (41.416, -0.5) -> (42.166, -1.799)
  line L537 (41.416, -3.0981) -> (39.916, -3.0981)
  line L538 (39.916, -0.5) -> (41.416, -0.5)
  line L539 (41.416, 0.5) -> (39.916, 0.5)
  line L540 (39.916, 3.0981) -> (41.416, 3.0981)
  line L541 (42.25, 3.5981) -> (42.25, 0) construction
  line L542 (42.25, 0) -> (43, 1.299)
  line L543 (42.25, 3.5981) -> (43, 4.8971)
  line L544 (43, 2.299) -> (42.25, 3.5981)
  line L545 (43, 1.299) -> (43, 2.299) construction
  line L546 (44.5, 2.299) -> (43, 2.299)
  line L547 (43, 4.8971) -> (44.5, 4.8971)
  line L548 (43, 1.299) -> (44.5, 1.299)
  line L549 (44.5, 1.299) -> (45.25, 0)
  line L550 (45.25, 3.5981) -> (44.5, 2.299)
  line L551 (46.116, 0.5) -> (45.366, 1.799)
  line L552 (45.366, 1.799) -> (46.116, 3.0981)
  line L553 (44.5, 4.8971) -> (45.25, 3.5981)
  line L554 (45.25, 0) -> (44.5, -1.299)
  line L555 (44.5, -1.299) -> (43, -1.299)
  line L556 (43, -1.299) -> (42.25, 0)
  line L557 (43, -1.299) -> (43, -2.299) construction
  line L558 (43, -2.299) -> (44.5, -2.299)
  line L559 (46.116, -3.0981) -> (45.366, -1.799)
  line L560 (42.25, -3.5981) -> (43, -2.299)
  line L561 (44.5, -2.299) -> (45.25, -3.5981)
  line L562 (43, -4.8971) -> (42.25, -3.5981)
  line L563 (44.5, -4.8971) -> (43, -4.8971)
  line L564 (45.25, -3.5981) -> (44.5, -4.8971)
  line L565 (45.366, -1.799) -> (46.116, -0.5)
  line L566 (48.4821, 0) -> (47.616, 0.5) construction
  line L567 (47.616, -0.5) -> (48.4821, 0) construction
  line L568 (47.616, 3.0981) -> (48.366, 1.799)
  line L569 (48.366, 1.799) -> (47.616, 0.5)
  line L570 (48.366, -1.799) -> (47.616, -3.0981)
  line L571 (47.616, -0.5) -> (48.366, -1.799)
  line L572 (47.616, -3.0981) -> (46.116, -3.0981)
  line L573 (46.116, -0.5) -> (47.616, -0.5)
  line L574 (47.616, 0.5) -> (46.116, 0.5)
  line L575 (46.116, 3.0981) -> (47.616, 3.0981)
  line L576 (48.45, 3.5981) -> (48.45, 0) construction
  line L577 (48.45, 0) -> (49.2, 1.299)
  line L578 (48.45, 3.5981) -> (49.2, 4.8971)
  line L579 (49.2, 2.299) -> (48.45, 3.5981)
  line L580 (49.2, 1.299) -> (49.2, 2.299) construction
  line L581 (50.7, 2.299) -> (49.2, 2.299)
  line L582 (49.2, 4.8971) -> (50.7, 4.8971)
  line L583 (49.2, 1.299) -> (50.7, 1.299)
  line L584 (50.7, 1.299) -> (51.45, 0)
  line L585 (51.45, 3.5981) -> (50.7, 2.299)
  line L586 (52.316, 0.5) -> (51.566, 1.799)
  line L587 (51.566, 1.799) -> (52.316, 3.0981)
  line L588 (50.7, 4.8971) -> (51.45, 3.5981)
  line L589 (51.45, 0) -> (50.7, -1.299)
  line L590 (50.7, -1.299) -> (49.2, -1.299)
  line L591 (49.2, -1.299) -> (48.45, 0)
  line L592 (49.2, -1.299) -> (49.2, -2.299) construction
  line L593 (49.2, -2.299) -> (50.7, -2.299)
  line L594 (52.316, -3.0981) -> (51.566, -1.799)
  line L595 (48.45, -3.5981) -> (49.2, -2.299)
  line L596 (50.7, -2.299) -> (51.45, -3.5981)
  line L597 (49.2, -4.8971) -> (48.45, -3.5981)
  line L598 (50.7, -4.8971) -> (49.2, -4.8971)
  line L599 (51.45, -3.5981) -> (50.7, -4.8971)
  line L600 (51.566, -1.799) -> (52.316, -0.5)
  line L601 (54.6821, 0) -> (53.816, 0.5) construction
  line L602 (53.816, -0.5) -> (54.6821, 0) construction
  line L603 (53.816, 3.0981) -> (54.566, 1.799)
  line L604 (54.566, 1.799) -> (53.816, 0.5)
  line L605 (54.566, -1.799) -> (53.816, -3.0981)
  line L606 (53.816, -0.5) -> (54.566, -1.799)
  line L607 (53.816, -3.0981) -> (52.316, -3.0981)
  line L608 (52.316, -0.5) -> (53.816, -0.5)
  line L609 (53.816, 0.5) -> (52.316, 0.5)
  line L610 (52.316, 3.0981) -> (53.816, 3.0981)
  line L611 (54.65, 3.5981) -> (54.65, 0) construction
  line L612 (54.65, 0) -> (55.4, 1.299)
  line L613 (54.65, 3.5981) -> (55.4, 4.8971)
  line L614 (55.4, 2.299) -> (54.65, 3.5981)
  line L615 (55.4, 1.299) -> (55.4, 2.299) construction
  line L616 (56.9, 2.299) -> (55.4, 2.299)
  line L617 (55.4, 4.8971) -> (56.9, 4.8971)
  line L618 (55.4, 1.299) -> (56.9, 1.299)
  line L619 (56.9, 1.299) -> (57.65, 0)
  line L620 (57.65, 3.5981) -> (56.9, 2.299)
  line L621 (58.516, 0.5) -> (57.766, 1.799)
  line L622 (57.766, 1.799) -> (58.516, 3.0981)
  line L623 (56.9, 4.8971) -> (57.65, 3.5981)
  line L624 (57.65, 0) -> (56.9, -1.299)
  line L625 (56.9, -1.299) -> (55.4, -1.299)
  line L626 (55.4, -1.299) -> (54.65, 0)
  line L627 (55.4, -1.299) -> (55.4, -2.299) construction
  line L628 (55.4, -2.299) -> (56.9, -2.299)
  line L629 (58.516, -3.0981) -> (57.766, -1.799)
  line L630 (54.65, -3.5981) -> (55.4, -2.299)
  line L631 (56.9, -2.299) -> (57.65, -3.5981)
  line L632 (55.4, -4.8971) -> (54.65, -3.5981)
  line L633 (56.9, -4.8971) -> (55.4, -4.8971)
  line L634 (57.65, -3.5981) -> (56.9, -4.8971)
  line L635 (57.766, -1.799) -> (58.516, -0.5)
  line L636 (60.8821, 0) -> (60.016, 0.5) construction
  line L637 (60.016, -0.5) -> (60.8821, 0) construction
  line L638 (60.016, 3.0981) -> (60.766, 1.799)
  line L639 (60.766, 1.799) -> (60.016, 0.5)
  line L640 (60.766, -1.799) -> (60.016, -3.0981)
  line L641 (60.016, -0.5) -> (60.766, -1.799)
  line L642 (60.016, -3.0981) -> (58.516, -3.0981)
  line L643 (58.516, -0.5) -> (60.016, -0.5)
  line L644 (60.016, 0.5) -> (58.516, 0.5)
  line L645 (58.516, 3.0981) -> (60.016, 3.0981)
  point P0 (0, 0)
  point P1 (-71.75, 0)
  point P2 (-89.25, 0)
  point P3 (78.25, 0)
  point P4 (89.25, 0)
  point P5 (-49.25, 0)
  point P6 (-54.25, 0)
  point P7 (-49.25, 3.5981)
  point P8 (-46.134, 1.799)
  point P9 (-49.25, -3.5981)
  point P10 (-46.134, -1.799)
  point P11 (-43.05, 3.5981)
  point P12 (-43.05, 0)
  point P13 (-43.05, -3.5981)
  point P14 (-38.434, 1.799)
  point P15 (-39.934, -1.799)
  point P16 (-39.934, 1.799)
  point P17 (-36.85, 3.5981)
  point P18 (-36.85, 0)
  point P19 (-36.85, -3.5981)
  point P20 (-32.234, 1.799)
  point P21 (-33.734, -1.799)
  point P22 (-33.734, 1.799)
  point P23 (-30.65, 3.5981)
  point P24 (-30.65, 0)
  point P25 (-30.65, -3.5981)
  point P26 (-26.034, 1.799)
  point P27 (-27.534, -1.799)
  point P28 (-27.534, 1.799)
  point P29 (-24.45, 3.5981)
  point P30 (-24.45, 0)
  point P31 (-24.45, -3.5981)
  point P32 (-19.834, 1.799)
  point P33 (-21.334, -1.799)
  point P34 (-21.334, 1.799)
  point P35 (-18.25, 3.5981)
  point P36 (-18.25, 0)
  point P37 (-18.25, -3.5981)
  point P38 (-13.634, 1.799)
  point P39 (-15.134, -1.799)
  point P40 (-15.134, 1.799)
  point P41 (-12.05, 3.5981)
  point P42 (-12.05, 0)
  point P43 (-12.05, -3.5981)
  point P44 (-7.434, 1.799)
  point P45 (-8.934, -1.799)
  point P46 (-8.934, 1.799)
  point P47 (-5.85, 3.5981)
  point P48 (-5.85, 0)
  point P49 (-5.85, -3.5981)
  point P50 (-1.234, 1.799)
  point P51 (-2.734, -1.799)
  point P52 (-2.734, 1.799)
  point P53 (0.35, 3.5981)
  point P54 (0.35, 0)
  point P55 (0.35, -3.5981)
  point P56 (4.966, 1.799)
  point P57 (3.466, -1.799)
  point P58 (3.466, 1.799)
  point P59 (6.55, 3.5981)
  point P60 (6.55, 0)
  point P61 (6.55, -3.5981)
  point P62 (11.166, 1.799)
  point P63 (9.666, -1.799)
  point P64 (9.666, 1.799)
  point P65 (12.75, 3.5981)
  point P66 (12.75, 0)
  point P67 (12.75, -3.5981)
  point P68 (17.366, 1.799)
  point P69 (15.866, -1.799)
  point P70 (15.866, 1.799)
  point P71 (18.95, 3.5981)
  point P72 (18.95, 0)
  point P73 (18.95, -3.5981)
  point P74 (23.566, 1.799)
  point P75 (22.066, -1.799)
  point P76 (22.066, 1.799)
  point P77 (25.15, 3.5981)
  point P78 (25.15, 0)
  point P79 (25.15, -3.5981)
  point P80 (29.766, 1.799)
  point P81 (28.266, -1.799)
  point P82 (28.266, 1.799)
  point P83 (31.35, 3.5981)
  point P84 (31.35, 0)
  point P85 (31.35, -3.5981)
  point P86 (35.966, 1.799)
  point P87 (34.466, -1.799)
  point P88 (34.466, 1.799)
  point P89 (37.55, 3.5981)
  point P90 (37.55, 0)
  point P91 (37.55, -3.5981)
  point P92 (42.166, 1.799)
  point P93 (40.666, -1.799)
  point P94 (40.666, 1.799)
  point P95 (43.75, 3.5981)
  point P96 (43.75, 0)
  point P97 (43.75, -3.5981)
  point P98 (48.366, 1.799)
  point P99 (46.866, -1.799)
  point P100 (46.866, 1.799)
  point P101 (49.95, 3.5981)
  point P102 (49.95, 0)
  point P103 (49.95, -3.5981)
  point P104 (54.566, 1.799)
  point P105 (53.066, -1.799)
  point P106 (53.066, 1.799)
  point P107 (56.15, 3.5981)
  point P108 (56.15, 0)
  point P109 (56.15, -3.5981)
  point P110 (60.766, 1.799)
  point P111 (59.266, -1.799)
  point P112 (59.266, 1.799)
  dimension "d1" = 12
  dimension "d3" = 23
  dimension "d4" = 10
  dimension "d5" = 150
  dimension "d6" = 3
  dimension "d7" = 5
  dimension "d8" = 3
  dimension "d9" = 1
  dimension "d10" = 1
  dimension "d11" = 1
  dimension "d12" = 1
  dimension "d13" = 1
  dimension "d14" = 1
  dimension "d24" = 6.2
  constraints: 1296 end point, 19 point on line, 18 coincident, 11 point on circle, 9 tangent, 8 equal length, 7 parallel, 6 horizontal, 6 midpoint, 4 centre point, 3 perpendicular, 2 collinear, 1 vertical, 1306 other
  measures "d1" distance of L0.end L1.end
  measures "d3" distance of L6.start L6.end
  measures "d4" distance of L9.end L9.start
  measures "d5" distance of point (78.25, 0) point (-71.75, 0)
  measures "d6" distance of L14.end L12.start
  measures "d7" distance of point (-54.25, 0) point (-49.25, 0)
  measures "d8" distance of L18.start L20.end
  measures "d9" distance between parallel lines of L16 L19
  measures "d10" distance of L18.end L26.end
  measures "d11" distance of L16.end L26.end
  measures "d12" distance of L39.end L12.end
  measures "d13" distance of L34.end L12.end
  measures "d14" distance of L39.end L34.end
  measures "d24" distance of L50.end L51.end
extrude "Extrusion1" add sketch "Sketch2" along normal mid plane 3 contours L0 A1 L2 A0 | L0 A2 L2 A1 | L0 A3 L2 A2
sketch "Sketch3" plane through (0, 0, -1.5) normal (0, 0, -1) x (-1, 0, 0)
  arc A0 (83.25, -6) -> (83.25, 6) centre (83.25, 0) ccw projected
  line L0 (60.25, 0) -> (83.25, 0) construction
  line L1 (-78.25, 0) -> (89.25, 0) construction
  point P0 (0, 0)
  point P1 (71.75, 0)
  dimension "d31" = 23
  dimension "d32" = 150
  constraints: 4 end point, 2 horizontal, 1 coincident, 1 midpoint, 1 point on circle
  measures "d31" distance of L0.end L0.start
  measures "d32" distance of point (71.75, 0) L1.start
hole "Hole1" at (78.25, 0, -1.5) at (-60.25, 0, -1.5) at (-83.25, 0, -1.5) direction (0, 0, 1) diameter 4.5 end through all clearance for "Socket Head Cap Screw" size "M4" standard "Ansi Metric M Profile"
hole "Hole2" at (-71.75, 0, -1.5) direction (0, 0, 1) diameter 5.5 end through all clearance for "Socket Head Cap Screw" size "M5" standard "Ansi Metric M Profile"
body "Solid1"
